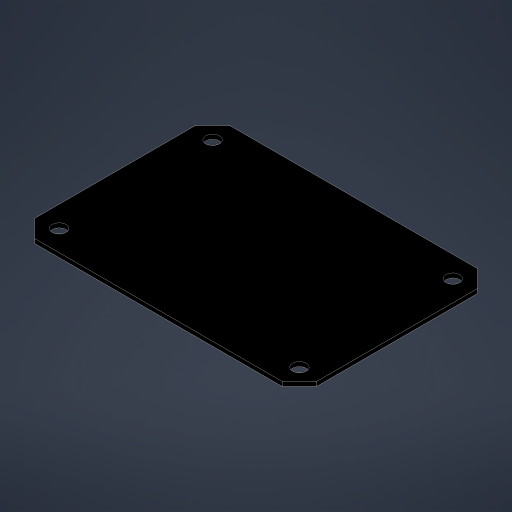
# Autodesk Inventor part: ShootPCB
Saved by Autodesk Inventor 2023 (Build 270158000, 158)
## iProperties
Created: 2023-03-13
Part Number: ShootPCB
Material: Generic
Document SubType Name: Modeling
Designer: Elias Braun
Density: 1 g/cm^3
Appearance: Default
Author: Elias Braun
Autodesk Inventor part; units mm, degrees
ref_plane "YZ Plane" through (0, 0, 0) normal (1, 0, 0) x (0, 1, 0)
ref_plane "XZ Plane" through (0, 0, 0) normal (0, 1, 0) x (-1, 0, 0)
ref_plane "XY Plane" through (0, 0, 0) normal (0, 0, 1) x (1, 0, 0)
sketch "Sketch1" plane through (0, 0, 0) normal (0, 1, 0) x (-1, 0, 0)
  line L0 (28.5, 22.5) -> (-28.5, 22.5)
  line L1 (-32.5, 18.5) -> (-32.5, -18.5)
  line L2 (-28.5, -22.5) -> (28.5, -22.5)
  line L3 (32.5, -18.5) -> (32.5, 18.5)
  line L4 (32.5, -18.5) -> (28.5, -22.5)
  line L5 (-28.5, -22.5) -> (-32.5, -18.5)
  line L6 (-32.5, 18.5) -> (-28.5, 22.5)
  line L7 (28.5, 22.5) -> (32.5, 18.5)
  line L8 (30.5, -20.5) -> (27.6716, -17.6716) construction
  line L9 (-30.5, -20.5) -> (-27.6716, -17.6716) construction
  line L10 (30.5, 20.5) -> (27.6716, 17.6716) construction
  line L11 (-30.5, 20.5) -> (-27.6716, 17.6716) construction
  circle A0 centre (27.6716, -17.6716) radius 1.6
  circle A1 centre (-27.6716, -17.6716) radius 1.6
  circle A2 centre (-27.6716, 17.6716) radius 1.6
  circle A3 centre (27.6716, 17.6716) radius 1.6
  point P0 (0, 0)
  point P1 (32.5, 22.5)
  point P2 (-32.5, 22.5)
  point P3 (-32.5, -22.5)
  point P4 (32.5, -22.5)
  dimension "d0" = 65
  dimension "d1" = 45
  dimension "d2" = 4
  dimension "d3" = 4
  dimension "d4" = 4
  dimension "d5" = 4
  dimension "d6" = 4
  dimension "d7" = 4
  dimension "d8" = 4
  dimension "d9" = 4
  dimension "d10" = 4
  dimension "d11" = 4
  dimension "d12" = 4
  dimension "d13" = 4
  dimension "d14" = 3.2
  dimension "d15" = 3.2
  dimension "d16" = 3.2
  dimension "d17" = 3.2
  constraints: 24 end point, 8 point on line, 4 centre point, 4 coincident, 4 midpoint, 2 parallel, 1 horizontal, 1 perpendicular
  measures "d0" distance of point (32.5, 22.5) point (-32.5, 22.5)
  measures "d1" distance of point (-32.5, -22.5) point (-32.5, 22.5)
  measures "d2" distance of L3.start point (32.5, -22.5)
  measures "d3" distance of L2.end point (32.5, -22.5)
  measures "d4" distance of L2.start point (-32.5, -22.5)
  measures "d5" distance of L1.end point (-32.5, -22.5)
  measures "d6" distance of L1.start point (-32.5, 22.5)
  measures "d7" distance of L0.end point (-32.5, 22.5)
  measures "d8" distance of L0.start point (32.5, 22.5)
  measures "d9" distance of L3.end point (32.5, 22.5)
  measures "d10" distance of L8.start L8.end
  measures "d11" distance of L9.start L9.end
  measures "d12" distance of L10.start L10.end
  measures "d13" distance of L11.start L11.end
  measures "d14" diameter of A0
  measures "d15" diameter of A1
  measures "d16" diameter of A2
  measures "d17" diameter of A3
extrude "Extrusion1" add sketch "Sketch1" along normal blind 1
sketch "Sketch2" plane through (0, 1, 0) normal (0, 1, 0) x (1, 0, 0)
  circle A0 centre (-27.6716, -17.6716) radius 2.8
  circle A1 centre (-27.6716, 17.6716) radius 2.8
  circle A2 centre (27.6716, 17.6716) radius 2.8
  circle A3 centre (27.6716, -17.6716) radius 2.8
  point P0 (0, 0)
  dimension "d20" = 5.6
  dimension "d21" = 5.6
  dimension "d22" = 5.6
  dimension "d23" = 5.6
  constraints: 4 centre point, 4 coincident
  measures "d20" diameter of A0
  measures "d21" diameter of A1
  measures "d22" diameter of A2
  measures "d23" diameter of A3
equation "\"d3\" = d2"
equation "\"d4\" = d2"
equation "\"d5\" = d4"
equation "\"d6\" = d2"
equation "\"d7\" = d6"
equation "\"d8\" = d2"
equation "\"d9\" = d8"
body "Solid1"
